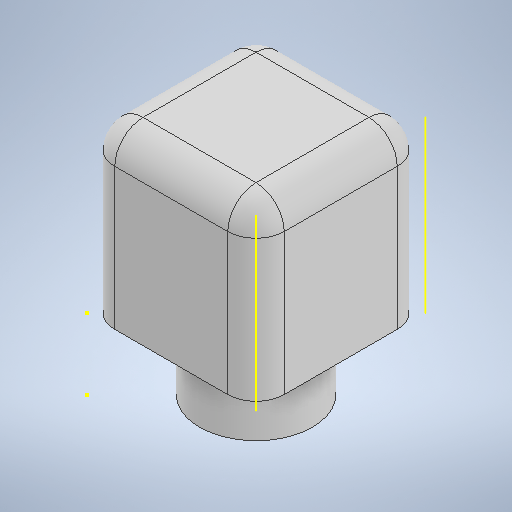
# Autodesk Inventor part: CONECTOR R-F
Saved by Autodesk Inventor 2025.2 (Build 292293000, 293)
## iProperties
Created: 2025-05-14
Part Number: CONECTOR R-F
Material: Genérico
Document SubType Name: Modeling
Designer: marce
Density: 1 g/cm^3
Appearance: Padrão
Author: marce
Autodesk Inventor part; units mm, degrees
ref_plane "YZ Plane" through (0, 0, 0) normal (1, 0, 0) x (0, 1, 0)
ref_plane "XZ Plane" through (0, 0, 0) normal (0, 1, 0) x (-1, 0, 0)
ref_plane "XY Plane" through (0, 0, 0) normal (0, 0, 1) x (1, 0, 0)
sketch "Esboço1" plane through (0, 0, 0) normal (1, 0, 0) x (0, 1, 0)
  line L0 (0, 0) -> (6, 0)
  line L1 (6, 0) -> (6, -6)
  line L2 (6, -6) -> (0, -6)
  line L3 (0, -6) -> (0, 0)
  dimension "d0" = 6
  dimension "d1" = 6
  constraints: 8 end point, 2 parallel, 1 horizontal, 1 perpendicular
  measures "d0" distance of L1.end L2.end
  measures "d1" distance of L0.end L1.end
extrude "Extrusão1" add sketch "Esboço1" along normal blind 6
sketch "Esboço2" plane through (0, 0, 0) normal (0, 0, 1) x (1, 0, 0)
  point P0 (0, 0)
sketch "Esboço3" plane through (6, 0, 0) normal (1, 0, 0) x (0, 0, -1)
  line L0 (0, 6) -> (0, 0) projected
  line L1 (6, 0) -> (6, 6) projected
sketch "Esboço4" plane through (0, 0, -6) normal (0, -1, 0) x (1, 0, 0)
  line L0 (0, 0) -> (0, 6) projected
  line L1 (6, 0) -> (6, 6) projected
  circle A0 centre (3, 3) radius 2
  dimension "d5" = 4
  constraints: 1 centre point
  measures "d5" diameter of A0
extrude "Extrusão2" add sketch "Esboço4" along normal blind 2.5
sketch "Esboço6" plane through (0, 0, 0) normal (-1, 0, 0) x (0, 0, 1)
  line L0 (-6, 6) -> (0, 6) projected
  line L1 (0, 0) -> (-6, 0) projected
  point P0 (-3, 3)
hole "Furo2" at (0, 3, -3) direction (1, 0, 0) diameter 3.242 depth 4 thread size "M4x0.7" class "6H" standard "ANSI Metric M Profile"
fillet "Arredondamento1" radius 1 1 edges at (6, 3, 0)
fillet "Arredondamento2" radius 1 3 edges at (6, 6, -3.5) (5.7071, 6, -0.2929) (2.5, 6, 0)
fillet "Arredondamento3" radius 1 3 edges at (0, 6, -3.5) (0, 5.7071, -0.2929) (0, 2.5, 0)
fillet "Arredondamento4" radius 1 5 edges at (0, 2.5, -6) (0.2929, 5.7071, -6) (3, 6, -6) (5.7071, 5.7071, -6) (6, 2.5, -6)
sketch "Esboço7" plane through (3, -2.5, -3) normal (0, -1, 0) x (1, 0, 0)
  point P0 (-3, 3)
sketch "Esboço8" plane through (3, -2.5, -3) normal (0, -1, 0) x (1, 0, 0)
  point P0 (-3, 3)
  point P1 (0, 0)
hole "Furo3" at (3, -2.5, -3) direction (0, 1, 0) diameter 2.459 depth 2 thread size "M3x0.5" class "6H" standard "ANSI Metric M Profile"
